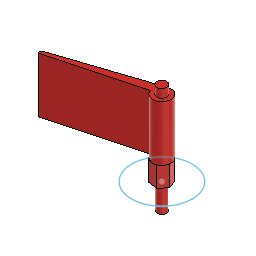
Poarta (Autodesk Fusion 360 design; units mm, degrees)
part number: 2026-06-02-22-05-38-321
Autodesk Fusion 360 part; units mm, degrees
note: some values were not read from the file. Set by a fixed rule: which sketch regions a step uses; which face or edge a step refers to.
sketch "Sketch1" plane through (0, 0, 0) normal (0, 0, 1) x (1, 0, 0)
  circle A0 centre (0, 0) radius 5.5
  line L0 (5.0888, -2.0866) -> (4.3514, 3.3638)
  line L1 (4.3514, 3.3638) -> (-0.7374, 5.4503)
  line L2 (-0.7374, 5.4503) -> (-5.0888, 2.0866)
  line L3 (-5.0888, 2.0866) -> (-4.3514, -3.3638)
  line L4 (-4.3514, -3.3638) -> (0.7374, -5.4503)
  line L5 (0.7374, -5.4503) -> (5.0888, -2.0866)
  line L6 (-60.0492, 0) -> (-60.086, 1.0214)
  line L7 (-59.145, 2.0557) -> (-0.3206, 5.4906)
  arc A1 (-59.145, 2.0557) -> (-60.086, 1.0214) centre (-59.0867, 1.0574) ccw
  circle A2 centre (0, 0) radius 2.75
  line L8 (-5.5, 0) -> (-60.0492, 0)
  point P0 (-60.1212, 1.9987)
  dimension "d1" = 11
  dimension "d2" = 55
  dimension "d3" = 2
  dimension "d4" = 1
  dimension "d7" = 5.5
  dimension "d59" = 5.4906
  dimension "d60" = 10.1777
  constraint coincident A0.centre A2.centre
  constraint coincident A0 L0.start
  constraint coincident A0 L7.end
  constraint tangent A0 L7
  constraint coincident P0 L6
  constraint coincident P0 L7
  constraint tangent L6 A1
  constraint tangent L7 A1
  constraint concentric A0 A2
  constraint coincident A0 L8.start
  constraint horizontal L8
  constraint horizontal A0.centre L6.start
  measures "d1" diameter of A0
  measures "d2" distance of L2.end L6.start
  measures "d3" distance of P0 L6.start
  measures "d4" radius of A1
  measures "d7" diameter of A2
  measures "d59" distance of L7.end L8
  measures "d60" horizontal distance of L0.start L2.end
extrude "Extrude1" add sketch "Sketch1" along normal blind 35 contours A0 L0 | A0 L1 | L0 L1 L2 L3 L4 L5 | A0 L5 | A0 L6 L7 A1 L8 | A0 L2 | A0 L4 | A0 L3 | A2
extrude "Extrude2" add sketch "Sketch1" against normal blind 10 contours L0 L1 L2 L3 L4 L5
extrude "Extrude3" add sketch "Sketch1" against normal blind 25 contours A2
move_body "Move1" bodies 1 to x (1, 0, 0) y (0, 1, 0) z (0, 0, 1) at (0, 0, 25)
move_body "Move2" bodies 1 to x (1, 0, 0) y (0, 1, 0) z (0, 0, 1) at (0, 0, 40)
extrude "Extrude4" cut 4 faces at (-21.6571, 3.1975, 65) (3.5158, -3.4529, 65) (4.9278, -0.0092, 65) (-2.4718, -4.263, 65) along direction (0, 0, 1) blind 1.2
move_body "Move3" bodies 1 to x (0.965926, 0.258819, 0) y (-0.258819, 0.965926, 0) z (0, 0, 1) at (0, 0, 0)
sketch "Sketch2" plane through (0, 0, 100) normal (0, 0, 1) x (-1, 0, 0)
  arc A0 (5.3126, 1.4235) -> (1.7308, -5.2206) centre (0, 0) ccw
  line L0 (1.7308, -5.2206) -> (57.6617, 13.3222)
  arc A1 (57.6617, 13.3222) -> (58.303, 14.5648) centre (57.347, 14.2714) ccw
  line L1 (58.303, 14.5648) -> (58.0031, 15.5419)
  line L2 (58.0031, 15.5419) -> (5.3126, 1.4235)
  circle A2 centre (0, 0) radius 3
  dimension "d300" = 6
  constraint concentric A0 A2
  measures "d300" diameter of A2
extrude "Extrude5" add sketch "Sketch2" along normal blind 5 contours A2
extrude "Extrude6" cut 4 faces at (-21.7467, -2.5167, 66.2) (4.2896, -2.4253, 66.2) (4.7622, 1.2665, 66.2) (0.0445, -4.9276, 66.2) along direction (0, 0, 1) blind 1
